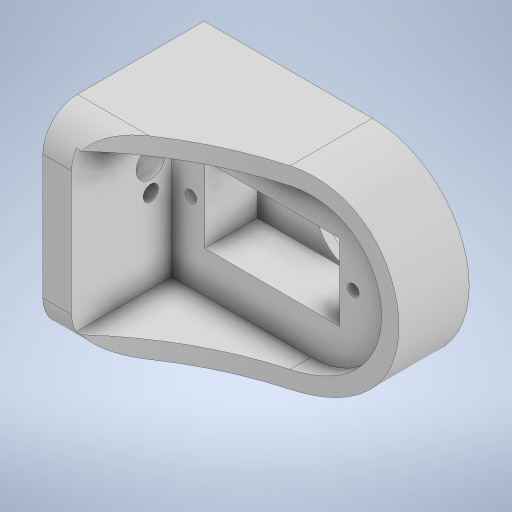
# Autodesk Inventor part: Final Arm 03
Saved by Autodesk Inventor 2024.1 (Build 281209000, 209)
## iProperties
Created: 2023-12-02
Part Number: Final Arm 03
Material: Generic
Document SubType Name: Modeling
Designer: vilas
Density: 1 g/cm^3
Appearance: Default
Author: vilas
Autodesk Inventor part; units mm, degrees
ref_plane "YZ Plane" through (0, 0, 0) normal (1, 0, 0) x (0, 1, 0)
ref_plane "XZ Plane" through (0, 0, 0) normal (0, 1, 0) x (-1, 0, 0)
ref_plane "XY Plane" through (0, 0, 0) normal (0, 0, 1) x (1, 0, 0)
sketch "Sketch1" plane through (0, 0, 0) normal (0, 0, 1) x (1, 0, 0)
  line L0 (0, 0) -> (115, 0)
  line L1 (115, 0) -> (115, 84)
  line L2 (115, 84) -> (0, 84)
  line L3 (0, 84) -> (0, 0)
  line L4 (115, 42) -> (0, 42) construction
  circle A0 centre (69, 42) radius 16.5
  arc A1 (73, 0) -> (73, 84) centre (73, 42) ccw
  dimension "d0" = 115
  dimension "d1" = 84
  dimension "d2" = 33
  dimension "d3" = 46
  constraints: 10 end point, 3 point on line, 3 tangent, 2 centre point, 2 midpoint, 2 parallel, 2 point on circle, 1 horizontal, 1 perpendicular
  measures "d0" distance of L2.end L1.end
  measures "d1" distance of L1.end L0.end
  measures "d2" diameter of A0
  measures "d3" distance from line of L1 A0.centre
extrude "Extrusion1" add sketch "Sketch1" along normal blind 70 contours L3 L2 A1 L0
sketch "Sketch2" plane through (0, 0, 70) normal (0, 0, 1) x (1, 0, 0)
  arc A0 (73, 0) -> (73, 84) centre (73, 42) ccw projected
  line L0 (73, 84) -> (0, 84)
  line L1 (0, 84) -> (0, 0)
  line L2 (0, 0) -> (73, 0)
  arc A1 (73, 0) -> (73, 84) centre (73, 42) ccw
  line L3 (12.5, 76.5) -> (73, 76.5)
  arc A2 (73, 7.5) -> (73, 76.5) centre (73, 42) ccw
  line L4 (73, 7.5) -> (12.5, 7.5)
  line L5 (12.5, 76.5) -> (12.5, 7.5)
  dimension "d6" = 7.5
  dimension "d7" = 12.5
  constraints: 12 end point, 4 point on circle, 3 perpendicular, 3 tangent, 2 centre point, 1 horizontal
  measures "d6" distance between parallel lines of L0 L3
  measures "d7" distance between parallel lines of L5 L1
extrude "Extrusion2" cut sketch "Sketch2" against normal blind 43.3 contours L3 A2 L4 L5
sketch "Sketch3" plane through (0, 0, 0) normal (0, 1, 0) x (-1, 0, 0)
  line L0 (0, 0) -> (0, 70) construction
  line L1 (0, 30.5) -> (-115.317, 30.5) construction
  line L2 (-73, 0) -> (-115, 0) construction
  line L3 (-73, 0) -> (0, 0) construction
  line L4 (-12.5, 0) -> (-12.5, 70) construction
  line L5 (-107.817, 30.5) -> (-107.817, 0) construction
  arc A0 (-115.317, 30.5) -> (-12.5, 70) centre (-111.567, 174.3032) ccw
  line L6 (-12.5, 70) -> (-115.317, 70)
  line L7 (-115.317, 30.5) -> (-115.317, 70)
  dimension "d10" = 30.5
  dimension "d11" = 12.5
  dimension "d12" = 7.5
  constraints: 10 end point, 4 point on line, 3 point on circle, 2 horizontal, 2 vertical, 1 centre point, 1 perpendicular
  measures "d10" distance between parallel lines of L2 L1
  measures "d11" distance between parallel lines of L4 L0
  measures "d12" distance from line of L1.end L5
extrude "Extrusion3" cut sketch "Sketch3" along normal through all
fillet "Fillet1" radius 15 2 edges at (6.25, 0, 70) (6.25, 84, 70)
sketch "Sketch4" plane through (12.5, 7.5, 26.7) normal (1, 0, 0) x (0, 0, -1)
  line L0 (-9.0174, -7.5) -> (-28.3, -7.5) construction
  line L1 (-9, -7.5) -> (-9, 76.5) construction
  line L2 (26.7, 76.5) -> (-28.3, 76.5) construction
  line L3 (0, 0) -> (0, 69) construction
  circle A0 centre (-9, 47.5) radius 6.35
  circle A1 centre (-9, 58.9) radius 3.3
  circle A2 centre (-9, 36.1) radius 3.3
  point P0 (26.7, -7.5)
  dimension "d16" = 9
  dimension "d17" = 12.7
  dimension "d18" = 29
  dimension "d19" = 6.6
  dimension "d20" = 11.4
  dimension "d21" = 6.6
  dimension "d22" = 11.4
  constraints: 5 point on line, 3 centre point, 2 end point, 1 vertical
  measures "d16" distance between parallel lines of L3 L1
  measures "d17" diameter of A0
  measures "d18" distance of L1.end A0.centre
  measures "d19" diameter of A1
  measures "d20" distance of A1.centre A0.centre
  measures "d21" diameter of A2
  measures "d22" distance of A0.centre A2.centre
extrude "Extrusion4" cut sketch "Sketch4" against normal through all
sketch "Sketch5" plane through (0, 0, 26.7) normal (0, 0, 1) x (1, 0, 0)
  circle A0 centre (69, 42) radius 16.5 construction
  line L0 (85.5, 42) -> (85.5, 58.5) construction
  line L1 (69, 58.5) -> (85.5, 58.5) construction
  line L2 (85.5, 58.5) -> (27, 58.5)
  line L3 (27, 58.5) -> (27, 25.5)
  line L4 (27, 25.5) -> (85.5, 25.5)
  line L5 (85.5, 25.5) -> (85.5, 58.5)
  point P0 (0, 0)
  dimension "d25" = 58.5
  constraints: 12 end point, 2 horizontal, 2 parallel, 2 point on circle, 1 perpendicular, 1 tangent, 1 vertical
  measures "d25" distance of L4.end L3.end
extrude "Extrusion5" cut sketch "Sketch5" against normal blind 22.8
sketch "Sketch6" plane through (0, 0, 26.7) normal (0, 0, 1) x (1, 0, 0)
  line L0 (27, 25.5) -> (27, 58.5) construction
  line L1 (27, 42) -> (12.5, 42) construction
  line L2 (12.5, 46.9) -> (12.5, 40.3) construction
  circle A0 centre (21, 42) radius 2.5
  line L3 (85.5, 25.5) -> (27, 25.5) construction
  line L4 (56.25, 25.5) -> (56.25, 58.5) construction
  circle A1 centre (91.5, 42) radius 2.5
  point P0 (0, 0)
  dimension "d28" = 5
  dimension "d29" = 6
  constraints: 4 end point, 2 centre point, 2 midpoint, 2 point on line, 1 horizontal, 1 symmetric about line, 1 vertical, 1 other
  measures "d28" diameter of A0
  measures "d29" distance from line of L0 A0.centre
extrude "Extrusion6" cut sketch "Sketch6" against normal blind 20.3
body "Solid1"
